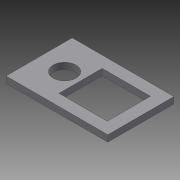
# Autodesk Inventor part: WoodD_Extruder_Side_Hole
Saved by Autodesk Inventor 2014 SP2 (Build 180246200, 246)
## iProperties
Created: 2014-09-30
Part Number: WoodD_Extruder_Side_Hole
Material: Generic
Document SubType Name: Modeling
Designer: ThatOtherGuy
Density: 1 g/cm^3
Appearance: Default
Author: ThatOtherGuy
Autodesk Inventor part; units mm, degrees
ref_plane "YZ Plane" through (0, 0, 0) normal (1, 0, 0) x (0, 1, 0)
ref_plane "XZ Plane" through (0, 0, 0) normal (0, 1, 0) x (-1, 0, 0)
ref_plane "XY Plane" through (0, 0, 0) normal (0, 0, 1) x (1, 0, 0)
sketch "Sketch1" plane through (0, 0, 0) normal (0, 0, 1) x (1, 0, 0)
  line L0 (0, 0) -> (100, 0)
  line L1 (100, 0) -> (100, 65)
  line L2 (100, 65) -> (0, 65)
  line L3 (0, 65) -> (0, 0)
  line L4 (88.25, 53.75) -> (40.75, 53.75)
  line L5 (40.75, 53.75) -> (40.75, 11.25)
  line L6 (40.75, 11.25) -> (88.25, 11.25)
  line L7 (88.25, 11.25) -> (88.25, 53.75)
  circle A0 centre (25, 32.5) radius 11.25
  point P0 (88.25, 32.5)
  point P1 (100, 32.5)
  point P2 (64.5, 53.75)
  dimension "d0" = 65
  dimension "d1" = 100
  dimension "d2" = 47.5
  dimension "d3" = 42.5
  dimension "d4" = 35.5
  dimension "d5" = 75
  dimension "d6" = 22.5
  constraints: 16 end point, 4 parallel, 3 midpoint, 2 horizontal, 2 horizontal alignment, 2 perpendicular, 1 centre point
  measures "d0" distance of L2.end L0.start
  measures "d1" distance of L0.start L0.end
  measures "d2" distance of L5.end L6.end
  measures "d3" distance of L4.end L5.end
  measures "d4" distance from line of L1 point (64.5, 53.75)
  measures "d5" distance from line of L1 A0.centre
  measures "d6" diameter of A0
extrude "Extrusion1" add sketch "Sketch1" along normal blind 6.35
equation "\"d7\" = THICKB"
equation "\"THICKA\" = 3.175"
equation "\"THICKB\" = 6.35"
equation "\"THICKC\" = 12.7"
body "Solid1"
